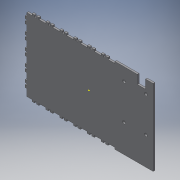
# Autodesk Inventor part: 3DprinterSideBracket_2.0
Saved by Autodesk Inventor 2016 (Build 200138000, 138)
## iProperties
Created: 2017-10-03
Part Number: 3DprinterSideBracket_2.0
Material: Generic
Document SubType Name: Modeling
Designer: jcj2131
Density: 1 g/cm^3
Appearance: Default
Author: jcj2131
Autodesk Inventor part; units mm, degrees
ref_plane "YZ Plane" through (0, 0, 0) normal (1, 0, 0) x (0, 1, 0)
ref_plane "XZ Plane" through (0, 0, 0) normal (0, 1, 0) x (-1, 0, 0)
ref_plane "XY Plane" through (0, 0, 0) normal (0, 0, 1) x (1, 0, 0)
sketch "Sketch1" plane through (0, 0, 0) normal (0, 0, 1) x (1, 0, 0)
  line L0 (-117.65, -70) -> (117.65, -70)
  line L1 (117.65, -70) -> (117.65, 70)
  line L2 (117.65, 70) -> (-117.65, 70)
  line L3 (-117.65, 70) -> (-117.65, -70)
  point P0 (0, 0)
  point P1 (-117.65, 0)
  point P2 (0, 70)
  dimension "d0" = 235.3
  dimension "d1" = 140
  constraints: 8 end point, 2 midpoint, 2 parallel, 1 horizontal, 1 horizontal alignment, 1 perpendicular, 1 vertical alignment
  measures "d0" distance of L1.end L2.end
  measures "d1" distance of L0.end L1.end
extrude "Extrusion1" add sketch "Sketch1" along normal blind 3.175
sketch "Sketch2" plane through (0, 0, 3.175) normal (0, 0, 1) x (1, 0, 0)
  circle A0 centre (104.15, 46.5) radius 2.75
  line L0 (117.65, 70) -> (-117.65, 70) projected
  line L1 (117.65, -70) -> (117.65, 70) projected
  circle A1 centre (64.15, 46.5) radius 2.75
  circle A2 centre (104.15, -18.5) radius 2.75
  circle A3 centre (64.15, -18.5) radius 2.75
  point P0 (0, 0)
  dimension "d4" = 23.5
  dimension "d5" = 13.5
  dimension "d6" = 5.5
  dimension "d7" = 5.5
  dimension "d8" = 23.5
  dimension "d9" = 40
  dimension "d10" = 5.5
  dimension "d11" = 13.5
  dimension "d12" = 65
  dimension "d13" = 5.5
  dimension "d14" = 40
  dimension "d15" = 65
  constraints: 4 centre point
  measures "d4" distance from line of L0 A0.centre
  measures "d5" distance from line of L1 A0.centre
  measures "d6" diameter of A0
  measures "d7" diameter of A1
  measures "d8" distance from line of L0 A1.centre
  measures "d9" distance of A0.centre A1.centre
  measures "d10" diameter of A2
  measures "d11" distance from line of L1 A2.centre
  measures "d12" distance of A2.centre A0.centre
  measures "d13" diameter of A3
  measures "d14" distance of A2.centre A3.centre
  measures "d15" distance of A1.centre A3.centre
extrude "Extrusion2" cut sketch "Sketch2" against normal through all
sketch "Sketch3" plane through (0, 0, 3.175) normal (0, 0, 1) x (1, 0, 0)
  line L0 (-117.65, 70) -> (-117.65, -70) projected
  line L1 (-117.65, -70) -> (-104.95, -70)
  line L2 (-104.95, -70) -> (-104.95, -66.825)
  line L3 (-104.95, -66.825) -> (-117.65, -66.825)
  line L4 (-117.65, -66.825) -> (-117.65, -70)
  point P0 (0, 0)
  dimension "d18" = 12.7
  dimension "d19" = 3.175
  constraints: 8 end point, 2 parallel, 1 horizontal, 1 perpendicular
  measures "d18" distance of L2.end L3.end
  measures "d19" distance of L1.end L2.end
extrude "Extrusion3" cut sketch "Sketch3" against normal through all
sketch "Sketch4" plane through (0, 0, 3.175) normal (0, 0, 1) x (1, 0, 0)
  line L0 (-104.95, -70) -> (117.65, -70) projected
  line L1 (-100.378, -70) -> (-96.822, -70)
  line L2 (-96.822, -70) -> (-96.822, -66.825)
  line L3 (-96.822, -66.825) -> (-100.378, -66.825)
  line L4 (-100.378, -66.825) -> (-100.378, -70)
  line L5 (-104.95, -66.825) -> (-104.95, -70) projected
  point P0 (0, 0)
  dimension "d22" = 3.556
  dimension "d23" = 3.175
  dimension "d24" = 4.572
  constraints: 8 end point, 2 parallel, 1 horizontal, 1 perpendicular, 1 point on line
  measures "d22" distance of L3.end L2.end
  measures "d23" distance of L1.end L2.end
  measures "d24" distance between parallel lines of L5 L4
extrude "Extrusion4" cut sketch "Sketch4" against normal through all
pattern_linear "Rectangular Pattern1" count 6 spacing 25.4 along (1, 0, 0) of "Extrusion3", "Extrusion4"
sketch "Sketch5" plane through (0, 0, 3.175) normal (0, 0, 1) x (1, 0, 0)
  line L0 (-82.65, -45) -> (81.35, -45)
  line L1 (81.35, -45) -> (81.35, 55)
  line L2 (81.35, 55) -> (-82.65, 55)
  line L3 (-82.65, 55) -> (-82.65, -45)
  line L4 (117.65, 70) -> (-117.65, 70) projected
  line L5 (-117.65, 70) -> (-117.65, -66.825) projected
  point P0 (0, 0)
  dimension "d30" = 164
  dimension "d31" = 100
  dimension "d32" = 15
  dimension "d33" = 35
  constraints: 8 end point, 2 parallel, 1 horizontal, 1 perpendicular
  measures "d30" distance of L1.end L2.end
  measures "d31" distance of L2.end L0.start
  measures "d32" distance between parallel lines of L4 L2
  measures "d33" distance between parallel lines of L5 L3
extrude "Extrusion5" [suppressed]
sketch "Sketch6" plane through (0, 0, 3.175) normal (0, 0, 1) x (1, 0, 0)
  circle A0 centre (-195.0968, -60.6866) radius 1.6
  line L0 (-190.0468, 40.3134) -> (-190.0468, -59.6866) projected
  line L1 (-26.0468, -59.6866) -> (-190.0468, -59.6866) projected
  circle A1 centre (-195.0968, 41.3134) radius 1.6
  line L2 (-190.0468, 40.3134) -> (-26.0468, 40.3134) projected
  circle A2 centre (-20.9968, 41.3134) radius 1.6
  line L3 (-26.0468, 40.3134) -> (-26.0468, -59.6866) projected
  circle A3 centre (-20.9968, -60.6866) radius 1.6
  point P0 (0, 0)
  dimension "d36" = 3.2
  dimension "d37" = 5.05
  dimension "d38" = 1
  dimension "d39" = 3.2
  dimension "d40" = 1
  dimension "d41" = 5.05
  dimension "d42" = 3.2
  dimension "d43" = 1
  dimension "d44" = 5.05
  dimension "d45" = 3.2
  dimension "d46" = 1
  dimension "d47" = 5.05
  constraints: 4 centre point
  measures "d36" diameter of A0
  measures "d37" distance from line of L0 A0.centre
  measures "d38" distance from line of L1 A0.centre
  measures "d39" diameter of A1
  measures "d40" distance from line of L2 A1.centre
  measures "d41" distance from line of L0 A1.centre
  measures "d42" diameter of A2
  measures "d43" distance from line of L2 A2.centre
  measures "d44" distance from line of L3 A2.centre
  measures "d45" diameter of A3
  measures "d46" distance from line of L1 A3.centre
  measures "d47" distance from line of L3 A3.centre
extrude "Extrusion6" [suppressed]
sketch "Sketch7" plane through (0, 0, 3.175) normal (0, 0, 1) x (1, 0, 0)
  line L0 (-117.65, 70) -> (-117.65, -66.825) projected
  line L1 (-117.65, -54.125) -> (-111.3, -54.125)
  line L2 (-111.3, -54.125) -> (-111.3, -41.425)
  line L3 (-111.3, -41.425) -> (-117.65, -41.425)
  line L4 (-117.65, -41.425) -> (-117.65, -54.125)
  line L5 (-117.65, -66.825) -> (-104.95, -66.825) projected
  point P0 (0, 0)
  dimension "d50" = 6.35
  dimension "d51" = 12.7
  dimension "d52" = 12.7
  constraints: 8 end point, 2 parallel, 1 horizontal, 1 perpendicular, 1 point on line
  measures "d50" distance of L3.end L2.end
  measures "d51" distance of L1.end L2.end
  measures "d52" distance between parallel lines of L5 L1
extrude "Extrusion7" [suppressed]
sketch "Sketch8" plane through (0, 0, 3.175) normal (0, 0, 1) x (1, 0, 0)
  line L0 (-148.4968, -45.6366) -> (-148.4968, -32.9366) projected
  line L1 (-148.4968, -41.0646) -> (-145.9568, -41.0646)
  line L2 (-145.9568, -41.0646) -> (-145.9568, -37.5086)
  line L3 (-145.9568, -37.5086) -> (-148.4968, -37.5086)
  line L4 (-148.4968, -37.5086) -> (-148.4968, -41.0646)
  line L5 (-154.8468, -32.9366) -> (-148.4968, -32.9366) projected
  point P0 (0, 0)
  dimension "d55" = 3.556
  dimension "d56" = 4.572
  dimension "d57" = 2.54
  constraints: 8 end point, 2 parallel, 1 horizontal, 1 perpendicular, 1 point on line
  measures "d55" distance of L1.end L2.end
  measures "d56" distance between parallel lines of L5 L3
  measures "d57" distance of L1.start L1.end
extrude "Extrusion8" [suppressed]
sketch "Sketch9" plane through (0, 0, 3.175) normal (0, 0, 1) x (1, 0, 0)
  line L0 (-145.9568, -43.2553) -> (-143.1786, -43.2553)
  line L1 (-143.1786, -43.2553) -> (-143.1786, -35.3178)
  line L2 (-143.1786, -35.3178) -> (-145.9568, -35.3178)
  line L3 (-145.9568, -35.3178) -> (-145.9568, -43.2553)
  line L4 (-145.9568, -37.5086) -> (-145.9568, -41.0646) projected
  line L5 (-117.65, 70) -> (-117.65, -66.825) projected
  line L6 (-117.65, -66.825) -> (-104.95, -66.825) projected
  line L7 (-104.95, -66.825) -> (-104.95, -70) projected
  line L8 (-104.95, -70) -> (-100.378, -70) projected
  line L9 (-100.378, -70) -> (-100.378, -66.825) projected
  line L10 (-100.378, -66.825) -> (-96.822, -66.825) projected
  line L11 (-96.822, -66.825) -> (-96.822, -70) projected
  line L12 (-96.822, -70) -> (-92.25, -70) projected
  line L13 (-92.25, -70) -> (-92.25, -66.825) projected
  line L14 (-92.25, -66.825) -> (-79.55, -66.825) projected
  line L15 (-79.55, -66.825) -> (-79.55, -70) projected
  line L16 (-79.55, -70) -> (-74.978, -70) projected
  line L17 (-74.978, -70) -> (-74.978, -66.825) projected
  line L18 (-74.978, -66.825) -> (-71.422, -66.825) projected
  line L19 (-71.422, -66.825) -> (-71.422, -70) projected
  line L20 (-71.422, -70) -> (-66.85, -70) projected
  line L21 (-66.85, -70) -> (-66.85, -66.825) projected
  line L22 (-66.85, -66.825) -> (-54.15, -66.825) projected
  line L23 (-54.15, -66.825) -> (-54.15, -70) projected
  line L24 (-54.15, -70) -> (-49.578, -70) projected
  line L25 (-49.578, -70) -> (-49.578, -66.825) projected
  line L26 (-49.578, -66.825) -> (-46.022, -66.825) projected
  line L27 (-46.022, -66.825) -> (-46.022, -70) projected
  line L28 (-46.022, -70) -> (-41.45, -70) projected
  line L29 (-41.45, -70) -> (-41.45, -66.825) projected
  line L30 (-41.45, -66.825) -> (-28.75, -66.825) projected
  line L31 (-28.75, -66.825) -> (-28.75, -70) projected
  line L32 (-28.75, -70) -> (-24.178, -70) projected
  line L33 (-24.178, -70) -> (-24.178, -66.825) projected
  line L34 (-24.178, -66.825) -> (-20.622, -66.825) projected
  line L35 (-20.622, -66.825) -> (-20.622, -70) projected
  line L36 (-20.622, -70) -> (-16.05, -70) projected
  line L37 (-16.05, -70) -> (-16.05, -66.825) projected
  line L38 (-16.05, -66.825) -> (-3.35, -66.825) projected
  line L39 (-3.35, -66.825) -> (-3.35, -70) projected
  line L40 (-3.35, -70) -> (1.222, -70) projected
  line L41 (1.222, -70) -> (1.222, -66.825) projected
  line L42 (1.222, -66.825) -> (4.778, -66.825) projected
  line L43 (4.778, -66.825) -> (4.778, -70) projected
  line L44 (4.778, -70) -> (9.35, -70) projected
  line L45 (9.35, -70) -> (9.35, -66.825) projected
  line L46 (9.35, -66.825) -> (22.05, -66.825) projected
  line L47 (22.05, -66.825) -> (22.05, -70) projected
  line L48 (22.05, -70) -> (26.622, -70) projected
  line L49 (26.622, -70) -> (26.622, -66.825) projected
  line L50 (26.622, -66.825) -> (30.178, -66.825) projected
  line L51 (30.178, -66.825) -> (30.178, -70) projected
  line L52 (117.65, -70) -> (117.65, 70) projected
  line L53 (117.65, 70) -> (-117.65, 70) projected
  circle A0 centre (104.15, -18.5) radius 2.75 projected
  circle A1 centre (104.15, 46.5) radius 2.75 projected
  circle A2 centre (64.15, 46.5) radius 2.75 projected
  circle A3 centre (64.15, -18.5) radius 2.75 projected
  line L54 (30.178, -70) -> (117.65, -70) projected
  point P0 (0, 0)
  dimension "d60" = 2.7781
  dimension "d61" = 7.9375
  constraints: 8 end point, 2 parallel, 1 horizontal, 1 perpendicular
  measures "d60" distance of L1.end L2.end
  measures "d61" distance of L0.end L1.end
extrude "Extrusion9" [suppressed]
sketch "Sketch10" plane through (0, 0, 3.175) normal (0, 0, 1) x (1, 0, 0)
  line L0 (-143.1786, -41.0643) -> (-102.41, -41.0643)
  line L1 (-102.41, -41.0643) -> (-102.41, -37.5088)
  line L2 (-102.41, -37.5088) -> (-143.1786, -37.5088)
  line L3 (-143.1786, -37.5088) -> (-143.1786, -41.0643)
  line L4 (-145.9568, -35.3178) -> (-143.1786, -35.3178) projected
  line L5 (-143.1786, -43.2553) -> (-145.9568, -43.2553) projected
  line L6 (-143.1786, -35.3178) -> (-143.1786, -43.2553) projected
  line L7 (-117.65, 70) -> (-117.65, -66.825) projected
  point P0 (0, 0)
  point P1 (-154.8468, -45.6366)
  point P2 (-117.65, -66.825)
  dimension "d65" = 2.191
  dimension "d66" = 2.191
  dimension "d67" = 0
  dimension "d68" = 15.24
  constraints: 8 end point, 2 parallel, 1 horizontal, 1 perpendicular, 1 other
  measures "d65" distance between parallel lines of L4 L2
  measures "d66" distance between parallel lines of L5 L0
  measures "d67" distance between parallel lines of L6 L3
extrude "Extrusion10" [suppressed]
sketch "Sketch11" plane through (0, 0, 3.175) normal (0, 0, 1) x (1, 0, 0)
  line L0 (-117.65, 70) -> (-117.65, -66.825) projected
  line L1 (-117.65, -66.825) -> (-114.475, -66.825)
  line L2 (-114.475, -66.825) -> (-114.475, -54.125)
  line L3 (-114.475, -54.125) -> (-117.65, -54.125)
  line L4 (-117.65, -54.125) -> (-117.65, -66.825)
  point P0 (0, 0)
  dimension "d71" = 3.175
  dimension "d72" = 12.7
  constraints: 8 end point, 2 parallel, 1 horizontal, 1 perpendicular
  measures "d71" distance of L2.end L3.end
  measures "d72" distance of L1.end L2.end
extrude "Extrusion11" cut sketch "Sketch11" against normal through all
sketch "Sketch12" plane through (0, 0, 3.175) normal (0, 0, 1) x (1, 0, 0)
  line L0 (-117.65, 70) -> (-117.65, -54.125) projected
  line L1 (-117.65, -49.5276) -> (-114.475, -49.5276)
  line L2 (-114.475, -49.5276) -> (-114.475, -46.0224)
  line L3 (-114.475, -46.0224) -> (-117.65, -46.0224)
  line L4 (-117.65, -46.0224) -> (-117.65, -49.5276)
  line L5 (-114.475, -54.125) -> (-117.65, -54.125) projected
  point P0 (0, 0)
  dimension "d75" = 3.5052
  dimension "d76" = 3.175
  dimension "d77" = 4.5974
  constraints: 8 end point, 2 parallel, 1 horizontal, 1 perpendicular, 1 point on line
  measures "d75" distance of L1.end L2.end
  measures "d76" distance of L2.end L3.end
  measures "d77" distance between parallel lines of L5 L1
extrude "Extrusion12" cut sketch "Sketch12" against normal through all
pattern_linear "Rectangular Pattern2" count 5 spacing 25.4 along (0, 1, 0) of "Extrusion11", "Extrusion12"
sketch "Sketch13" plane through (0, 0, 3.175) normal (0, 0, 1) x (1, 0, 0)
  line L0 (117.65, 70) -> (-117.65, 70) projected
  line L1 (-117.65, 70) -> (-111.3, 70)
  line L2 (-111.3, 70) -> (-111.3, 34.775)
  line L3 (-111.3, 34.775) -> (-117.65, 34.775)
  line L4 (-117.65, 34.775) -> (-117.65, 70)
  line L5 (-117.65, 30.1776) -> (-114.475, 30.1776) projected
  point P0 (0, 0)
  dimension "d83" = 6.35
  dimension "d84" = 4.5974
  constraints: 8 end point, 2 parallel, 1 horizontal, 1 perpendicular
  measures "d83" distance of L2.end L3.end
  measures "d84" distance between parallel lines of L3 L5
extrude "Extrusion13" [suppressed]
sketch "Sketch14" plane through (-190.0468, -59.6866, 6.35) normal (0, 1, 0) x (1, 0, 0)
  point P0 (190.0468, 6.35)
sketch "Sketch15" plane through (0, 0, 3.175) normal (0, 0, 1) x (1, 0, 0)
  point P0 (0, 0)
sketch "Sketch16" plane through (0, 0, 3.175) normal (0, 0, 1) x (1, 0, 0)
  line L0 (117.65, 70) -> (-117.65, 70) projected
  line L1 (88.65, 70) -> (103.65, 70)
  line L2 (103.65, 70) -> (103.65, 53.9306)
  line L3 (103.65, 53.9306) -> (88.65, 53.9306)
  line L4 (88.65, 53.9306) -> (88.65, 70)
  line L5 (117.65, -70) -> (117.65, 70) projected
  point P0 (0, 0)
  point P1 (-148.4968, 55.3134)
  dimension "d87" = 15
  dimension "d88" = 14
  constraints: 8 end point, 2 parallel, 1 horizontal, 1 perpendicular, 2 other
  measures "d87" distance of L2.end L3.end
  measures "d88" distance between parallel lines of L5 L2
extrude "Extrusion14" cut sketch "Sketch16" against normal through all
sketch "Sketch17" plane through (0, 0, 3.175) normal (0, 0, 1) x (1, 0, 0)
  line L0 (88.65, 70) -> (-117.65, 70) projected
  line L1 (-117.65, 70) -> (-114.475, 70)
  line L2 (-114.475, 70) -> (-114.475, 60.175)
  line L3 (-114.475, 60.175) -> (-117.65, 60.175)
  line L4 (-117.65, 60.175) -> (-117.65, 70)
  line L5 (-114.475, 55.5776) -> (-117.65, 55.5776) projected
  point P0 (0, 0)
  dimension "d91" = 3.175
  dimension "d92" = 4.5974
  constraints: 8 end point, 2 parallel, 1 horizontal, 1 perpendicular
  measures "d91" distance of L2.end L3.end
  measures "d92" distance between parallel lines of L5 L3
extrude "Extrusion15" cut sketch "Sketch17" against normal through all
sketch "Sketch18" plane through (0, 0, 3.175) normal (0, 0, 1) x (1, 0, 0)
  line L0 (30.178, -70) -> (117.65, -70) projected
  line L1 (34.75, -70) -> (47.45, -70)
  line L2 (47.45, -70) -> (47.45, -66.825)
  line L3 (47.45, -66.825) -> (34.75, -66.825)
  line L4 (34.75, -66.825) -> (34.75, -70)
  line L5 (30.178, -66.825) -> (30.178, -70) projected
  point P0 (0, 0)
  dimension "d95" = 3.175
  dimension "d96" = 12.7
  dimension "d97" = 4.572
  constraints: 8 end point, 2 parallel, 1 horizontal, 1 perpendicular, 1 point on line
  measures "d95" distance of L1.end L2.end
  measures "d96" distance of L2.end L3.end
  measures "d97" distance between parallel lines of L5 L4
extrude "Extrusion16" cut sketch "Sketch18" against normal through all
mirror "Mirror1" about plane through (0, 0, 0) normal (0, 1, 0) of "Rectangular Pattern1", "Extrusion3", "Extrusion4", "Extrusion16"
body "Solid1"
